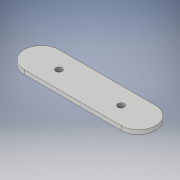
# Autodesk Inventor part: FrameBracket
Saved by Autodesk Inventor 2018 (Build 220112000, 112)
## iProperties
Created: 2019-10-18
Part Number: FrameBracket
Material: Generic
Document SubType Name: Modeling
Designer: anirudh
Density: 1 g/cm^3
Appearance: Default
Author: anirudh
Autodesk Inventor part; units mm, degrees
ref_plane "YZ Plane" through (0, 0, 0) normal (1, 0, 0) x (0, 1, 0)
ref_plane "XZ Plane" through (0, 0, 0) normal (0, 1, 0) x (-1, 0, 0)
ref_plane "XY Plane" through (0, 0, 0) normal (0, 0, 1) x (1, 0, 0)
sketch "Sketch1" plane through (0, 0, 0) normal (0, 1, 0) x (-1, 0, 0)
  circle A0 centre (-105.9111, 9.525) radius 1.75
  circle A1 centre (-71.9005, 9.525) radius 1.75
  circle A2 centre (-105.9111, 9.525) radius 1.75
  circle A3 centre (-71.9005, 9.525) radius 1.75
  line L0 (-62.3755, 0) -> (-115.4361, 0)
  line L1 (-62.3755, 19.05) -> (-115.4361, 19.05)
  arc A4 (-115.4361, 19.05) -> (-115.4361, 0) centre (-115.4361, 9.525) ccw
  arc A5 (-62.3755, 0) -> (-62.3755, 19.05) centre (-62.3755, 9.525) ccw
  point P0 (0, 0)
  constraints: 6 centre point, 4 end point, 4 point on circle, 2 concentric, 1 coincident
extrude "Extrusion1" add sketch "Sketch1" along normal blind 2.286
body "Solid1"
